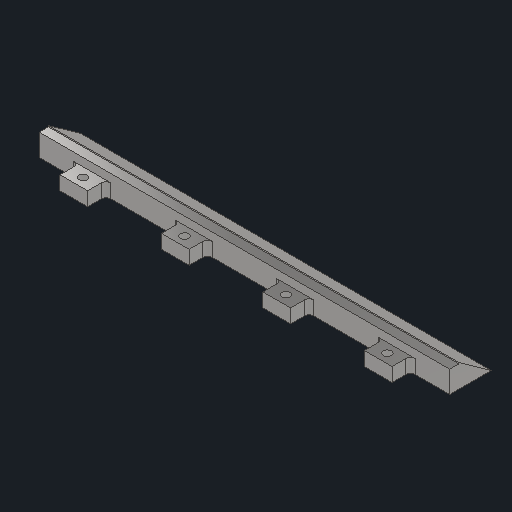
# Autodesk Inventor part: plog
Saved by Autodesk Inventor 2023 (Build 270158000, 158)
## iProperties
Created: 2024-04-10
Part Number: plog
Material: Steel, Alloy
Document SubType Name: Modeling
Designer: szymo
Density: 7.73 g/cm^3
Appearance: Semi-Polished
Mass: 164.375 g
Surface Area: 102.615 cm^2
Volume: 21.2646 cm^3
Author: szymo
Autodesk Inventor part; units mm, degrees
ref_plane "YZ Plane" through (0, 0, 0) normal (1, 0, 0) x (0, 1, 0)
ref_plane "XZ Plane" through (0, 0, 0) normal (0, 1, 0) x (-1, 0, 0)
ref_plane "XY Plane" through (0, 0, 0) normal (0, 0, 1) x (1, 0, 0)
sketch "Sketch3" plane through (0, 0, 0) normal (1, 0, 0) x (0, 1, 0)
  line L0 (0, 0) -> (10, 0)
  line L1 (10, 0) -> (10, -14)
  line L2 (10, -14) -> (0, -14)
  line L3 (0, -14) -> (0, 0)
  line L4 (10, 0) -> (0, -14)
  line L5 (6, 0) -> (0, 0)
  line L6 (0, 0) -> (0, 12)
  line L7 (0, 12) -> (6, 12)
  line L8 (6, 12) -> (6, 0)
  line L9 (9.5, 0) -> (6, 0)
  line L10 (6, 0) -> (6, 4)
  line L11 (6, 4) -> (9.5, 4)
  line L12 (9.5, 4) -> (9.5, 0)
  dimension "d30" = 12
  dimension "d31" = 6
  dimension "d63" = 10
  dimension "d74" = 0.5
  dimension "d75" = 4
  dimension "d76" = 3.5
  dimension "d141" = 35.538
  dimension "d142" = 14
  constraints: 26 end point, 6 parallel, 4 point on line, 3 horizontal, 3 perpendicular
  measures "d30" distance of L5.end L6.end
  measures "d31" distance of L6.end L7.end
  measures "d63" distance of L1.end L2.end
  measures "d74" distance between parallel lines of L1 L12
  measures "d75" distance between parallel lines of L11 L0
  measures "d76" distance of L10.end L11.end
  measures "d141" angle of L4 L3
  measures "d142" distance of L0.end L1.end
extrude "Extrusion2" add sketch "Sketch3" along normal blind 178 contours L6 L7 L8 L0 | L0 L4 L3 | L8 L11 L12 L0
sketch "Sketch10" plane through (0, 0, -14) normal (0, -1, 0) x (1, 0, 0)
  line L0 (0, 18) -> (0, 26) projected
  line L1 (0, 26) -> (178, 26) projected
  line L2 (178, 18) -> (178, 26) projected
  line L3 (0, 18) -> (178, 18) projected
  line L4 (0, 14) -> (0, 18) projected
  line L5 (0, 18) -> (17, 18)
  line L6 (17, 18) -> (17, 26)
  line L7 (17, 26) -> (0, 26)
  line L8 (0, 26) -> (0, 18)
  line L9 (0, 18) -> (178, 18) projected
  line L10 (178, 26) -> (161, 26)
  line L11 (161, 26) -> (161, 18)
  line L12 (161, 18) -> (178, 18)
  line L13 (178, 18) -> (178, 26)
  line L14 (17, 26) -> (29, 26)
  line L15 (29, 26) -> (29, 18)
  line L16 (29, 18) -> (17, 18)
  line L17 (17, 18) -> (17, 26)
  line L18 (61, 26) -> (73, 26)
  line L19 (73, 26) -> (73, 18)
  line L20 (73, 18) -> (61, 18)
  line L21 (61, 18) -> (61, 26)
  line L22 (105, 26) -> (117, 26)
  line L23 (117, 26) -> (117, 18)
  line L24 (117, 18) -> (105, 18)
  line L25 (105, 18) -> (105, 26)
  line L26 (149, 26) -> (161, 26)
  line L27 (161, 26) -> (161, 18)
  line L28 (161, 18) -> (149, 18)
  line L29 (149, 18) -> (149, 26)
  line L30 (17, 26) -> (29, 18)
  line L31 (29, 26) -> (17, 18)
  line L32 (61, 26) -> (73, 18)
  line L33 (73, 26) -> (61, 18)
  line L34 (105, 26) -> (117, 18)
  line L35 (117, 26) -> (105, 18)
  line L36 (149, 26) -> (161, 18)
  line L37 (161, 26) -> (149, 18)
  point P0 (105, 18)
  point P1 (23, 22)
  point P2 (67, 22)
  point P3 (111, 22)
  point P4 (155, 22)
  dimension "d118" = 17
  dimension "d119" = 17
  dimension "d120" = 12
  dimension "d121" = 12
  dimension "d122" = 12
  dimension "d123" = 12
  dimension "d124" = 0
  dimension "d125" = 0
  dimension "d126" = 32
  dimension "d129" = 32
  dimension "d130" = 32
  constraints: 64 end point, 12 parallel, 10 point on line, 6 horizontal, 6 perpendicular, 4 midpoint
  measures "d118" distance of L7.end L6.end
  measures "d119" distance of L12.end L11.end
  measures "d120" distance of L15.end L16.end
  measures "d121" distance of L19.end L20.end
  measures "d122" distance of L23.end L24.end
  measures "d123" distance of L27.end L28.end
  measures "d124" distance between parallel lines of L6 L17
  measures "d125" distance between parallel lines of L27 L11
  measures "d126" distance between parallel lines of L23 L29
  measures "d129" distance between parallel lines of L15 L21
  measures "d130" distance between parallel lines of L19 L25
extrude "Extrusion5" cut sketch "Sketch10" against normal up to next contours L0 L1 L6 L3 | L15 L1 L21 L3 | L19 L1 L25 L3 | L23 L1 L29 L3 | L11 L1 L2 L3
hole "Hole4" at (23, 0, 8) at (67, 0, 8) at (111, 0, 8) at (155, 0, 8) direction (0, 1, 0) diameter 3.6 end through all countersink diameter 6.5 countersink angle 90 clearance for "Countersunk Flat Head Screw ISO 2009/7046" size "M3" standard "ISO"
fillet "Fillet2" radius 2 8 edges at (17, 3, 4) (29, 3, 4) (61, 3, 4) (73, 3, 4) (105, 3, 4) (117, 3, 4) (149, 3, 4) (161, 3, 4)
equation "\"d126\" = d130"
equation "\"d129\" = d130"
body "Solid2"
